Autodesk Fusion 360 part; units mm, degrees
(part 5 of 5)
  spline S37 degree 5 poles (28.0678, 2.6304) (28.0819, 2.6317) (28.1102, 2.634) (28.1526, 2.6363) (28.2093, 2.6371) (28.2803, 2.6353) (28.3513, 2.6314) (28.4224, 2.6261) (28.4935, 2.6201) (28.5647, 2.6137) (28.6359, 2.6067) (28.7071, 2.5991) (28.7783, 2.5906) (28.8495, 2.5811) (28.9207, 2.5705) (28.9919, 2.559) (29.0631, 2.5467) (29.1343, 2.5337) (29.2055, 2.5201) (29.2767, 2.5059) (29.3478, 2.4912) (29.419, 2.4759) (29.4901, 2.46) (29.5612, 2.4434) (29.6322, 2.4261) (29.7033, 2.4083) (29.7743, 2.3899) (29.8453, 2.3709) (29.9162, 2.3515) (29.9871, 2.3314) (30.058, 2.3109) (30.1288, 2.2899) (30.1996, 2.2683) (30.2704, 2.2463) (30.3411, 2.2237) (30.4117, 2.2006) (30.4824, 2.1771) (30.5529, 2.153) (30.6235, 2.1285) (30.6939, 2.1035) (30.7644, 2.0781) (30.8347, 2.0522) (30.905, 2.0259) (30.9753, 1.9991) (31.0455, 1.9718) (31.1156, 1.9441) (31.1857, 1.916) (31.2558, 1.8874) (31.3257, 1.8584) (31.3956, 1.829) (31.4655, 1.7992) (31.5352, 1.7689) (31.6049, 1.7383) (31.6746, 1.7072) (31.7442, 1.6757) (31.8137, 1.6438) (31.8831, 1.6115) (31.9524, 1.5788) (32.0217, 1.5457) (32.0909, 1.5122) (32.1601, 1.4784) (32.2291, 1.4441) (32.2981, 1.4094) (32.367, 1.3744) (32.4359, 1.339) (32.5046, 1.3032) (32.5733, 1.267) (32.6419, 1.2305) (32.7104, 1.1936) (32.7788, 1.1563) (32.8471, 1.1186) (32.9017, 1.0882) (32.9427, 1.0652) (32.9699, 1.0499) (32.9835, 1.0421) knots 0 0 0 0 0 0 0.01428571 0.02857143 0.04285714 0.05714286 0.07142857 0.08571429 0.1 0.11428571 0.12857143 0.14285714 0.15714286 0.17142857 0.18571429 0.2 0.21428571 0.22857143 0.24285714 0.25714286 0.27142857 0.28571429 0.3 0.31428571 0.32857143 0.34285714 0.35714286 0.37142857 0.38571429 0.4 0.41428571 0.42857143 0.44285714 0.45714286 0.47142857 0.48571429 0.5 0.51428571 0.52857143 0.54285714 0.55714286 0.57142857 0.58571429 0.6 0.61428571 0.62857143 0.64285714 0.65714286 0.67142857 0.68571429 0.7 0.71428571 0.72857143 0.74285714 0.75714286 0.77142857 0.78571429 0.8 0.81428571 0.82857143 0.84285714 0.85714286 0.87142857 0.88571429 0.9 0.91428571 0.92857143 0.94285714 0.95714286 0.97142857 0.98571429 1 1 1 1 1 1
  line L37 (28.0678, 2.6304) -> (27.7691, 2.6026)
  arc A74 (26.0521, 3.9455) -> (27.7691, 2.6026) centre (27.6217, 4.1832) ccw
  arc A75 (26.0521, 3.9455) -> (25.9963, 4.2981) centre (0, 0) ccw
  arc A76 (27.2142, 6.1059) -> (25.9963, 4.2981) centre (27.5625, 4.5571) ccw
  line L38 (27.2142, 6.1059) -> (27.5069, 6.1717)
  spline S38 degree 5 poles (27.5069, 6.1717) (27.5207, 6.1748) (27.5483, 6.1814) (27.5894, 6.1924) (27.6436, 6.2091) (27.7105, 6.2328) (27.7768, 6.2585) (27.8428, 6.2854) (27.9086, 6.3131) (27.9743, 6.3412) (28.0399, 6.3698) (28.1052, 6.3991) (28.1703, 6.4291) (28.2351, 6.4602) (28.2996, 6.4923) (28.3637, 6.5252) (28.4276, 6.5589) (28.4913, 6.5933) (28.5548, 6.6282) (28.6182, 6.6637) (28.6813, 6.6997) (28.7442, 6.7362) (28.8069, 6.7734) (28.8694, 6.8111) (28.9317, 6.8495) (28.9937, 6.8884) (29.0556, 6.9278) (29.1172, 6.9678) (29.1786, 7.0083) (29.2399, 7.0492) (29.301, 7.0906) (29.3618, 7.1325) (29.4225, 7.1749) (29.483, 7.2177) (29.5432, 7.261) (29.6033, 7.3048) (29.6632, 7.3491) (29.7229, 7.3937) (29.7824, 7.4388) (29.8417, 7.4844) (29.9008, 7.5303) (29.9597, 7.5767) (30.0185, 7.6235) (30.077, 7.6707) (30.1353, 7.7183) (30.1935, 7.7663) (30.2515, 7.8147) (30.3092, 7.8635) (30.3668, 7.9127) (30.4242, 7.9623) (30.4814, 8.0122) (30.5384, 8.0626) (30.5952, 8.1133) (30.6519, 8.1644) (30.7083, 8.2158) (30.7645, 8.2676) (30.8206, 8.3198) (30.8765, 8.3723) (30.9321, 8.4252) (30.9876, 8.4784) (31.0429, 8.532) (31.098, 8.5859) (31.1529, 8.6402) (31.2076, 8.6948) (31.2621, 8.7498) (31.3164, 8.8051) (31.3706, 8.8607) (31.4245, 8.9166) (31.4783, 8.9729) (31.5318, 9.0295) (31.5852, 9.0864) (31.6277, 9.1322) (31.6595, 9.1667) (31.6807, 9.1898) (31.6913, 9.2013) knots 0 0 0 0 0 0 0.01428571 0.02857143 0.04285714 0.05714286 0.07142857 0.08571429 0.1 0.11428571 0.12857143 0.14285714 0.15714286 0.17142857 0.18571429 0.2 0.21428571 0.22857143 0.24285714 0.25714286 0.27142857 0.28571429 0.3 0.31428571 0.32857143 0.34285714 0.35714286 0.37142857 0.38571429 0.4 0.41428571 0.42857143 0.44285714 0.45714286 0.47142857 0.48571429 0.5 0.51428571 0.52857143 0.54285714 0.55714286 0.57142857 0.58571429 0.6 0.61428571 0.62857143 0.64285714 0.65714286 0.67142857 0.68571429 0.7 0.71428571 0.72857143 0.74285714 0.75714286 0.77142857 0.78571429 0.8 0.81428571 0.82857143 0.84285714 0.85714286 0.87142857 0.88571429 0.9 0.91428571 0.92857143 0.94285714 0.95714286 0.97142857 0.98571429 1 1 1 1 1 1
  arc A77 (31.6913, 9.2013) -> (31.0472, 11.1836) centre (0, 0) ccw
  spline S39 degree 5 poles (25.8812, 11.1751) (25.8942, 11.1807) (25.9204, 11.1916) (25.9601, 11.2069) (26.0137, 11.2252) (26.0818, 11.2454) (26.1506, 11.2636) (26.2198, 11.2806) (26.2893, 11.2969) (26.359, 11.3128) (26.4288, 11.3281) (26.4989, 11.3429) (26.5692, 11.3568) (26.6399, 11.3697) (26.7109, 11.3817) (26.7822, 11.3928) (26.8537, 11.4031) (26.9254, 11.4127) (26.9973, 11.4218) (27.0694, 11.4303) (27.1416, 11.4383) (27.214, 11.4457) (27.2866, 11.4525) (27.3593, 11.4587) (27.4322, 11.4643) (27.5053, 11.4693) (27.5785, 11.4737) (27.6519, 11.4776) (27.7254, 11.481) (27.799, 11.4839) (27.8727, 11.4863) (27.9466, 11.4881) (28.0206, 11.4895) (28.0947, 11.4904) (28.1689, 11.4908) (28.2433, 11.4907) (28.3177, 11.4901) (28.3922, 11.489) (28.4669, 11.4875) (28.5416, 11.4855) (28.6165, 11.4831) (28.6914, 11.4802) (28.7664, 11.4769) (28.8415, 11.4731) (28.9167, 11.4689) (28.992, 11.4642) (29.0673, 11.4591) (29.1427, 11.4536) (29.2182, 11.4477) (29.2938, 11.4413) (29.3695, 11.4345) (29.4452, 11.4273) (29.5209, 11.4196) (29.5968, 11.4116) (29.6727, 11.4032) (29.7486, 11.3943) (29.8246, 11.385) (29.9007, 11.3754) (29.9768, 11.3653) (30.053, 11.3549) (30.1292, 11.344) (30.2055, 11.3328) (30.2818, 11.3211) (30.3582, 11.3091) (30.4346, 11.2967) (30.511, 11.2839) (30.5875, 11.2707) (30.664, 11.2572) (30.7406, 11.2432) (30.8172, 11.2289) (30.8938, 11.2142) (30.9551, 11.2022) (31.0011, 11.193) (31.0318, 11.1867) (31.0472, 11.1836) knots 0 0 0 0 0 0 0.01428571 0.02857143 0.04285714 0.05714286 0.07142857 0.08571429 0.1 0.11428571 0.12857143 0.14285714 0.15714286 0.17142857 0.18571429 0.2 0.21428571 0.22857143 0.24285714 0.25714286 0.27142857 0.28571429 0.3 0.31428571 0.32857143 0.34285714 0.35714286 0.37142857 0.38571429 0.4 0.41428571 0.42857143 0.44285714 0.45714286 0.47142857 0.48571429 0.5 0.51428571 0.52857143 0.54285714 0.55714286 0.57142857 0.58571429 0.6 0.61428571 0.62857143 0.64285714 0.65714286 0.67142857 0.68571429 0.7 0.71428571 0.72857143 0.74285714 0.75714286 0.77142857 0.78571429 0.8 0.81428571 0.82857143 0.84285714 0.85714286 0.87142857 0.88571429 0.9 0.91428571 0.92857143 0.94285714 0.95714286 0.97142857 0.98571429 1 1 1 1 1 1
  line L39 (25.8812, 11.1751) -> (25.6057, 11.0563)
  arc A78 (23.5578, 11.803) -> (25.6057, 11.0563) centre (24.9771, 12.5141) ccw
  arc A79 (23.5578, 11.803) -> (23.3957, 12.1211) centre (0, 0) ccw
  circle A80 centre (0, 0) radius 26.3492
  constraint coincident A1.centre A3.centre
  constraint coincident A15.end A80
extrude "Extrude4" add sketch "Sketch2 (2)" along normal blind 3.75 contours A3 A7 A11 A15 A19 A23 A27 A31 A35 A39 A43 A47 A51 A55 A59 A63 A67 A71 A75 A79 A80 in component "Spur Gear (20 teeth)"
sketch "Sketch3 (2)" plane through (0, 0, 6.25) normal (0, 0, 1) x (-1, 0, 0)
  circle A0 centre (0, 0) radius 26.3492
  circle A1 centre (0, 0) radius 2.75
  circle A2 centre (0, 0) radius 5
  line L0 (-1.8715, 2.015) -> (1.8715, 2.015)
  line L1 (-1.8715, -2.015) -> (1.8715, -2.015)
  dimension "d13" = 5.5
  dimension "d14" = 10
  constraint concentric A0 A1
  constraint concentric A0 A2
  constraint coincident A1 L0.start
  constraint coincident A1 L0.end
  constraint horizontal L0
  constraint coincident A1 L1.start
  constraint coincident A1 L1.end
  constraint parallel L0 L1
  measures "d13" diameter of A1
  measures "d14" diameter of A2
extrude "Extrude5" add sketch "Sketch3 (2)" along normal blind 10 contours A1 L0 | A1 L1 | A2 in component "Spur Gear (20 teeth)"
component "Spur Gear (20 teeth)" placed x (1, 0, 0) y (0, 1, 0) z (0, 0, 1) at (0, 0, 0)
